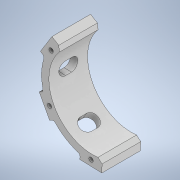
# Autodesk Inventor part: end_holder_3
Saved by Autodesk Inventor 2020 (Build 240168000, 168)
## iProperties
Created: 2020-11-16
Part Number: end_holder_3
Material: Generic
Document SubType Name: Modeling
Designer: Shuang Peng
Density: 1 g/cm^3
Appearance: Default
Author: Shuang Peng
Autodesk Inventor part; units mm, degrees
ref_plane "Work Plane1" through (0, 0, 0) normal (0, 0, 1) x (1, 0, 0)
sketch "Sketch1" plane through (0, 0, 0) normal (0, 0, 1) x (1, 0, 0)
  line L0 (-114.7595, -23.8164) -> (-86.516, -0.3214) projected
  arc A0 (-83.238, -1.9261) -> (-86.516, -0.3214) centre (-85.2369, -1.8589) ccw projected
  arc A1 (-83.238, -1.9261) -> (-80.4978, -22.1613) centre (-22.2724, -3.9734) ccw projected
  arc A2 (-84.3159, -27.354) -> (-80.4978, -22.1613) centre (-84.3159, -23.354) ccw projected
  line L1 (-84.3159, -27.354) -> (-113.4805, -27.354) projected
  arc A3 (-114.7595, -23.8164) -> (-113.4805, -27.354) centre (-113.4805, -25.354) ccw projected
  circle A4 centre (71.296, -16.8454) radius 1.5 projected
  circle A5 centre (-18.8152, -59.8032) radius 1.5 projected
  circle A6 centre (-53.4562, -50.8504) radius 1.5 projected
  circle A7 centre (-60.8075, 36.5725) radius 1.5 projected
  circle A8 centre (-28.5162, 51.9811) radius 1.5 projected
  circle A9 centre (-9.173, 50.4079) radius 1.5 projected
  circle A10 centre (-44.8423, 47.6065) radius 1.5 projected
  circle A11 centre (-67.2628, -37.2117) radius 1.5 projected
  circle A12 centre (-38.1378, -57.9935) radius 1.5 projected
  circle A13 centre (45.81, -34.6909) radius 1.5 projected
  circle A14 centre (-22.2724, -3.9734) radius 24.5 projected
  line L2 (17.4995, 54.7179) -> (28.6687, 48.4472) projected
  line L3 (8.4026, 48.2499) -> (17.4995, 54.7179) projected
  arc A15 (6.5013, 48.0227) -> (8.4026, 48.2499) centre (7.2436, 49.8798) ccw projected
  line L4 (-7.3529, 53.5603) -> (6.5013, 48.0227) projected
  arc A16 (-7.3529, 53.5603) -> (-12.4241, 54.6417) centre (-22.2724, -3.9734) ccw projected
  line L5 (-12.5849, 53.6843) -> (-12.4241, 54.6417) projected
  arc A17 (-14.821, 52.0331) -> (-12.5849, 53.6843) centre (-14.5573, 54.0157) ccw projected
  arc A18 (-14.821, 52.0331) -> (-23.537, 52.5125) centre (-22.2724, -3.9734) ccw projected
  arc A19 (-25.5786, 54.3989) -> (-23.537, 52.5125) centre (-23.5818, 54.512) ccw projected
  line L6 (-25.6541, 55.7327) -> (-25.5786, 54.3989) projected
  arc A20 (-25.6541, 55.7327) -> (-31.8766, 55.0521) centre (-22.2724, -3.9734) ccw projected
  line L7 (-43.4677, 51.9463) -> (-31.8766, 55.0521) projected
  arc A21 (-43.4677, 51.9463) -> (-49.1968, 49.4245) centre (-22.2724, -3.9734) ccw projected
  line L8 (-48.5953, 48.2316) -> (-49.1968, 49.4245) projected
  arc A22 (-49.4201, 45.5771) -> (-48.5953, 48.2316) centre (-50.3811, 47.3311) ccw projected
  arc A23 (-49.4201, 45.5771) -> (-56.7287, 40.804) centre (-22.2724, -3.9734) ccw projected
  arc A24 (-59.4908, 41.1159) -> (-56.7287, 40.804) centre (-57.9484, 42.389) ccw projected
  line L9 (-60.1088, 41.8646) -> (-59.4908, 41.1159) projected
  arc A25 (-60.1088, 41.8646) -> (-63.9599, 38.3925) centre (-22.2724, -3.9734) ccw projected
  line L10 (-73.8637, 25.8129) -> (-63.9599, 38.3925) projected
  line L11 (-73.8637, 25.8129) -> (-144.5637, -33.0004) projected
  arc A26 (-144.5637, -33.0004) -> (-146.1648, -34.4172) centre (-122.1805, -59.9075) ccw projected
  arc A27 (-148.5912, -34.6592) -> (-146.1648, -34.4172) centre (-147.5353, -32.9607) ccw projected
  line L12 (-148.5912, -34.6592) -> (-150.0693, -33.7404) projected
  line L13 (-150.0693, -33.7404) -> (-157.9882, -46.4797) projected
  line L14 (-157.9882, -46.4797) -> (-156.5102, -47.3985) projected
  arc A28 (-155.6533, -49.6815) -> (-156.5102, -47.3985) centre (-157.566, -49.0971) ccw projected
  arc A29 (-155.6533, -49.6815) -> (-156.2478, -67.9334) centre (-122.1805, -59.9075) ccw projected
  arc A30 (-157.2515, -70.1557) -> (-156.2478, -67.9334) centre (-158.1945, -68.392) ccw projected
  line L15 (-157.2515, -70.1557) -> (-158.7862, -70.9764) projected
  line L16 (-158.7862, -70.9764) -> (-151.7131, -84.204) projected
  line L17 (-151.7131, -84.204) -> (-150.1784, -83.3834) projected
  arc A31 (-147.7729, -83.7828) -> (-150.1784, -83.3834) centre (-149.2353, -85.1471) ccw projected
  arc A32 (-147.7729, -83.7828) -> (-132.2635, -93.4236) centre (-122.1805, -59.9075) ccw projected
  arc A33 (-130.8408, -95.404) -> (-132.2635, -93.4236) centre (-132.8397, -95.3388) ccw projected
  line L18 (-130.8408, -95.404) -> (-130.8974, -97.1434) projected
  line L19 (-130.8974, -97.1434) -> (-115.9054, -97.6318) projected
  line L20 (-115.9054, -97.6318) -> (-115.8487, -95.8923) projected
  arc A34 (-114.3001, -94.0088) -> (-115.8487, -95.8923) centre (-113.8498, -95.9574) ccw projected
  arc A35 (-114.3001, -94.0088) -> (-111.5272, -93.2468) centre (-122.1805, -59.9075) ccw projected
  line L21 (-111.5272, -93.2468) -> (-17.5702, -63.2237) projected
  line L22 (-1.8974, -59.9532) -> (-17.5702, -63.2237) projected
  line L23 (-3.6226, -55.2133) -> (-1.8974, -59.9532) projected
  arc A36 (-2.4006, -52.6404) -> (-3.6226, -55.2133) centre (-1.7432, -54.5293) ccw projected
  line L24 (40.7711, -37.6143) -> (-2.4006, -52.6404) projected
  arc A37 (41.7759, -37.5336) -> (40.7711, -37.6143) centre (41.4286, -39.5032) ccw projected
  line L25 (49.1414, -38.8323) -> (41.7759, -37.5336) projected
  line L26 (49.5371, -36.5883) -> (49.1414, -38.8323) projected
  arc A38 (51.1536, -34.967) -> (49.5371, -36.5883) centre (51.5067, -36.9355) ccw projected
  arc A39 (51.1536, -34.967) -> (69.7278, -21.9611) centre (46.3856, -8.3913) ccw projected
  arc A40 (71.8042, -20.9967) -> (69.7278, -21.9611) centre (71.4569, -22.9663) ccw projected
  line L27 (74.0482, -21.3924) -> (71.8042, -20.9967) projected
  line L28 (78.128, 1.745) -> (74.0482, -21.3924) projected
  line L29 (78.128, 1.745) -> (69.8258, 3.2089) projected
  arc A41 (28.6687, 48.4472) -> (69.8258, 3.2089) centre (78.5082, 52.4493) ccw projected
  circle A42 centre (46.3856, -8.3913) radius 8 projected
  circle A43 centre (24.8362, 42.9855) radius 2.1 projected
  circle A44 centre (69.0444, -1.2227) radius 2.1 projected
  circle A45 centre (32.9741, 22.501) radius 2.1 projected
  circle A46 centre (48.56, 6.9152) radius 2.1 projected
  line L30 (61.5225, -11.0604) -> (64.993, -11.6723) projected
  arc A47 (66.5678, -14.1946) -> (64.993, -11.6723) centre (64.6457, -13.6419) ccw projected
  arc A48 (55.6053, -27.2592) -> (66.5678, -14.1946) centre (46.3856, -8.3913) ccw projected
  arc A49 (52.8479, -26.1463) -> (55.6053, -27.2592) centre (54.7273, -25.4622) ccw projected
  line L31 (52.8479, -26.1463) -> (51.6426, -22.8348) projected
  arc A50 (52.6012, -20.3753) -> (51.6426, -22.8348) centre (53.522, -22.1507) ccw projected
  arc A51 (52.6012, -20.3753) -> (59.2669, -12.4314) centre (46.3856, -8.3913) ccw projected
  arc A52 (61.5225, -11.0604) -> (59.2669, -12.4314) centre (61.1752, -13.03) ccw projected
  arc A53 (28.8077, -30.3754) -> (33.319, -18.6649) centre (-22.2724, -3.9734) ccw projected
  arc A54 (36.6892, -17.7843) -> (33.319, -18.6649) centre (35.2527, -19.1759) ccw projected
  arc A55 (36.6892, -17.7843) -> (42.4768, -21.313) centre (46.3856, -8.3913) ccw projected
  arc A56 (43.0588, -24.8558) -> (42.4768, -21.313) centre (41.8977, -23.2274) ccw projected
  line L32 (43.0588, -24.8558) -> (31.7455, -32.9222) projected
  arc A57 (28.8077, -30.3754) -> (31.7455, -32.9222) centre (30.5844, -31.2938) ccw projected
  arc A58 (36.3695, 11.8712) -> (41.3146, 7.2953) centre (78.5082, 52.4493) ccw projected
  arc A59 (40.8614, 3.9267) -> (41.3146, 7.2953) centre (40.043, 5.7516) ccw projected
  arc A60 (40.8614, 3.9267) -> (37.576, 1.8381) centre (46.3856, -8.3913) ccw projected
  arc A61 (34.2864, 3.1052) -> (37.576, 1.8381) centre (36.2709, 3.3536) ccw projected
  arc A62 (34.2864, 3.1052) -> (32.9898, 9.9939) centre (-22.2724, -3.9734) ccw projected
  arc A63 (36.3695, 11.8712) -> (32.9898, 9.9939) centre (34.9289, 10.4839) ccw projected
  circle A64 centre (-78.0027, -75.3364) radius 2 projected
  circle A65 centre (-110.6431, -14.2192) radius 2 projected
  circle A66 centre (-91.7471, -81.3441) radius 2 projected
  circle A67 centre (-123.1684, -22.4726) radius 2 projected
  circle A68 centre (-123.2712, -93.3897) radius 1.5 projected
  circle A69 centre (-150.6316, -42.2218) radius 1.5 projected
  circle A70 centre (-151.7223, -75.704) radius 1.5 projected
  circle A71 centre (-76.5892, -34.383) radius 2.05 projected
  circle A72 centre (-93.5857, -34.7301) radius 2.05 projected
  circle A73 centre (-85.7696, -48.6911) radius 2.05 projected
  line L33 (25.2192, -8.9275) -> (12.7605, -6.9639) projected
  arc A74 (10.2276, -3.9982) -> (12.7605, -6.9639) centre (13.2276, -4.0005) ccw projected
  arc A75 (10.2276, -3.9982) -> (9.854, 0.9403) centre (-22.2724, -3.9734) ccw projected
  arc A76 (12.117, 4.3104) -> (9.854, 0.9403) centre (12.8195, 1.3938) ccw projected
  line L34 (12.117, 4.3104) -> (24.3016, 7.2454) projected
  arc A77 (27.9589, 4.8477) -> (24.3016, 7.2454) centre (25.0042, 4.3289) ccw projected
  arc A78 (28.6837, -6.0885) -> (27.9589, 4.8477) centre (-22.2724, -3.9734) ccw projected
  arc A79 (25.2192, -8.9275) -> (28.6837, -6.0885) centre (25.6863, -5.9641) ccw projected
  line L35 (18.5933, -28.9733) -> (7.9021, -22.4328) projected
  arc A80 (6.7854, -18.53) -> (7.9021, -22.4328) centre (9.4676, -19.8737) ccw projected
  arc A81 (6.7854, -18.53) -> (8.6598, -13.9459) centre (-22.2724, -3.9734) ccw projected
  arc A82 (11.9821, -11.903) -> (8.6598, -13.9459) centre (11.515, -14.8664) ccw projected
  line L36 (11.9821, -11.903) -> (24.4408, -13.8666) projected
  arc A83 (26.8641, -17.6335) -> (24.4408, -13.8666) centre (23.9738, -16.83) ccw projected
  arc A84 (22.8108, -27.8167) -> (26.8641, -17.6335) centre (-22.2724, -3.9734) ccw projected
  arc A85 (18.5933, -28.9733) -> (22.8108, -27.8167) centre (20.1588, -26.4142) ccw projected
  line L37 (-4.4447, -43.3488) -> (-7.3459, -35.8081) projected
  arc A86 (-6.0439, -32.1316) -> (-7.3459, -35.8081) centre (-4.5459, -34.7308) ccw projected
  arc A87 (-6.0439, -32.1316) -> (-1.9539, -29.3388) centre (-22.2724, -3.9734) ccw projected
  arc A88 (2.0962, -29.6136) -> (-1.9539, -29.3388) centre (-0.0783, -31.6803) ccw projected
  line L38 (2.0962, -29.6136) -> (7.6236, -35.4294) projected
  arc A89 (7.3609, -39.808) -> (7.6236, -35.4294) centre (5.449, -37.4961) ccw projected
  arc A90 (-0.2222, -44.9128) -> (7.3609, -39.808) centre (-22.2724, -3.9734) ccw projected
  arc A91 (-4.4447, -43.3488) -> (-0.2222, -44.9128) centre (-1.6448, -42.2715) ccw projected
  line L39 (-23.3755, -47.3558) -> (-23.1715, -39.3349) projected
  arc A92 (-20.35, -36.4165) -> (-23.1715, -39.3349) centre (-20.1725, -39.4112) ccw projected
  arc A93 (-20.35, -36.4165) -> (-15.4428, -35.7477) centre (-22.2724, -3.9734) ccw projected
  arc A94 (-12.0124, -37.6034) -> (-15.4428, -35.7477) centre (-14.8123, -38.6807) ccw projected
  line L40 (-12.0124, -37.6034) -> (-9.1112, -45.1441) projected
  arc A95 (-11.1966, -49.135) -> (-9.1112, -45.1441) centre (-11.9112, -46.2214) ccw projected
  arc A96 (-20.2457, -50.4292) -> (-11.1966, -49.135) centre (-22.2724, -3.9734) ccw projected
  arc A97 (-23.3755, -47.3558) -> (-20.2457, -50.4292) centre (-20.3765, -47.432) ccw projected
  line L41 (-50.3087, -42.6252) -> (-42.3788, -32.8175) projected
  arc A98 (-38.5439, -32.1067) -> (-42.3788, -32.8175) centre (-40.0459, -34.7037) ccw projected
  arc A99 (-38.5439, -32.1067) -> (-34.0803, -34.2525) centre (-22.2724, -3.9734) ccw projected
  arc A100 (-32.2932, -37.8973) -> (-34.0803, -34.2525) centre (-35.1703, -37.0474) ccw projected
  line L42 (-32.2932, -37.8973) -> (-35.8437, -49.917) projected
  arc A101 (-39.7488, -51.8855) -> (-35.8437, -49.917) centre (-38.7208, -49.0672) ccw projected
  arc A102 (-49.5823, -47.0451) -> (-39.7488, -51.8855) centre (-22.2724, -3.9734) ccw projected
  arc A103 (-50.3087, -42.6252) -> (-49.5823, -47.0451) centre (-47.9758, -44.5114) ccw projected
  line L43 (-64.3558, -26.8641) -> (-53.346, -20.8755) projected
  arc A104 (-49.4077, -21.8598) -> (-53.346, -20.8755) centre (-51.9125, -23.5108) ccw projected
  arc A105 (-49.4077, -21.8598) -> (-46.3749, -25.7752) centre (-22.2724, -3.9734) ccw projected
  arc A106 (-46.2669, -29.6738) -> (-46.3749, -25.7752) centre (-48.5998, -27.7876) ccw projected
  line L44 (-46.2669, -29.6738) -> (-54.1968, -39.4816) projected
  arc A107 (-58.6707, -39.6968) -> (-54.1968, -39.4816) centre (-56.5296, -37.5954) ccw projected
  arc A108 (-65.463, -31.0949) -> (-58.6707, -39.6968) centre (-22.2724, -3.9734) ccw projected
  arc A109 (-64.3558, -26.8641) -> (-65.463, -31.0949) centre (-62.9223, -29.4995) ccw projected
  line L45 (-65.2864, 0.2751) -> (-57.3053, -0.9828) projected
  arc A110 (-54.7724, -3.9485) -> (-57.3053, -0.9828) centre (-57.7724, -3.9462) ccw projected
  arc A111 (-54.7724, -3.9485) -> (-54.3988, -8.887) centre (-22.2724, -3.9734) ccw projected
  arc A112 (-56.6618, -12.2571) -> (-54.3988, -8.887) centre (-57.3643, -9.3405) ccw projected
  line L46 (-56.6618, -12.2571) -> (-64.4621, -14.1361) projected
  arc A113 (-68.1227, -11.7192) -> (-64.4621, -14.1361) centre (-65.1646, -11.2195) ccw projected
  arc A114 (-68.7521, -2.5997) -> (-68.1227, -11.7192) centre (-22.2724, -3.9734) ccw projected
  arc A115 (-65.2864, 0.2751) -> (-68.7521, -2.5997) centre (-65.7534, -2.6883) ccw projected
  line L47 (-59.2911, 18.6731) -> (-52.4469, 14.4861) projected
  arc A116 (-51.3302, 10.5833) -> (-52.4469, 14.4861) centre (-54.0124, 11.927) ccw projected
  arc A117 (-51.3302, 10.5833) -> (-53.2046, 5.9991) centre (-22.2724, -3.9734) ccw projected
  arc A118 (-56.5269, 3.9563) -> (-53.2046, 5.9991) centre (-56.0599, 6.9197) ccw projected
  line L48 (-56.5269, 3.9563) -> (-64.5079, 5.2141) projected
  arc A119 (-66.9215, 9.0155) -> (-64.5079, 5.2141) centre (-64.0409, 8.1775) ccw projected
  arc A120 (-63.5177, 17.4994) -> (-66.9215, 9.0155) centre (-22.2724, -3.9734) ccw projected
  arc A121 (-59.2911, 18.6731) -> (-63.5177, 17.4994) centre (-60.8567, 16.114) ccw projected
  line L49 (-41.7278, 39.6327) -> (-37.199, 27.8613) projected
  arc A122 (-38.5009, 24.1849) -> (-37.199, 27.8613) centre (-39.9989, 26.7841) ccw projected
  arc A123 (-38.5009, 24.1849) -> (-42.5909, 21.3921) centre (-22.2724, -3.9734) ccw projected
  arc A124 (-46.641, 21.6668) -> (-42.5909, 21.3921) centre (-44.4665, 23.7336) ccw projected
  line L50 (-46.641, 21.6668) -> (-55.2752, 30.7515) projected
  arc A125 (-55.0274, 35.1177) -> (-55.2752, 30.7515) centre (-53.1006, 32.8182) ccw projected
  arc A126 (-45.9187, 41.2135) -> (-55.0274, 35.1177) centre (-22.2724, -3.9734) ccw projected
  arc A127 (-41.7278, 39.6327) -> (-45.9187, 41.2135) centre (-44.5277, 38.5555) ccw projected
  line L51 (-21.0547, 43.9173) -> (-21.3733, 31.3882) projected
  arc A128 (-24.1948, 28.4697) -> (-21.3733, 31.3882) centre (-24.3723, 31.4645) ccw projected
  arc A129 (-24.1948, 28.4697) -> (-29.1021, 27.8009) centre (-22.2724, -3.9734) ccw projected
  arc A130 (-32.5324, 29.6567) -> (-29.1021, 27.8009) centre (-29.7325, 30.7339) ccw projected
  line L52 (-32.5324, 29.6567) -> (-37.0613, 41.4281) projected
  arc A131 (-35.0106, 45.4102) -> (-37.0613, 41.4281) centre (-34.2613, 42.5053) ccw projected
  arc A132 (-24.1651, 46.9915) -> (-35.0106, 45.4102) centre (-22.2724, -3.9734) ccw projected
  arc A133 (-21.0547, 43.9173) -> (-24.1651, 46.9915) centre (-24.0537, 43.9936) ccw projected
  line L53 (5.7638, 34.6785) -> (-2.166, 24.8708) projected
  arc A134 (-6.0009, 24.16) -> (-2.166, 24.8708) centre (-4.4989, 26.757) ccw projected
  arc A135 (-6.0009, 24.16) -> (-10.4645, 26.3057) centre (-22.2724, -3.9734) ccw projected
  arc A136 (-12.2517, 29.9506) -> (-10.4645, 26.3057) centre (-9.3746, 29.1007) ccw projected
  line L54 (-12.2517, 29.9506) -> (-8.7012, 41.9703) projected
  arc A137 (-4.796, 43.9388) -> (-8.7012, 41.9703) centre (-5.8241, 41.1205) ccw projected
  arc A138 (5.0374, 39.0984) -> (-4.796, 43.9388) centre (-22.2724, -3.9734) ccw projected
  arc A139 (5.7638, 34.6785) -> (5.0374, 39.0984) centre (3.431, 36.5647) ccw projected
  circle A140 centre (18.7379, 18.9865) radius 2.05 projected
  circle A141 centre (5.6495, 11.6589) radius 2.05 projected
  arc A142 (-88.373, -68.9659) -> (-87.2274, -61.7195) centre (-122.1805, -59.9075) ccw projected
  arc A143 (-84.7539, -56.3391) -> (-87.2274, -61.7195) centre (-79.2381, -62.1337) ccw projected
  line L55 (-84.7539, -56.3391) -> (-72.896, -45.0519) projected
  arc A144 (-67.1926, -45.2429) -> (-72.896, -45.0519) centre (-70.1382, -47.9491) ccw projected
  arc A145 (-67.1926, -45.2429) -> (-52.2157, -57.1184) centre (-22.2724, -3.9734) ccw projected
  arc A146 (-52.5887, -60.766) -> (-52.2157, -57.1184) centre (-53.1975, -58.8609) ccw projected
  line L56 (-52.5887, -60.766) -> (-85.8324, -71.3887) projected
  arc A147 (-88.373, -68.9659) -> (-85.8324, -71.3887) centre (-86.4412, -69.4836) ccw projected
  arc A148 (-119.4703, -38.0751) -> (-123.464, -37.945) centre (-121.4642, -37.9192) ccw projected
  arc A149 (-100.218, -58.6239) -> (-119.4703, -38.0751) centre (-122.1805, -59.9075) ccw projected
  arc A150 (-100.3481, -62.6177) -> (-100.218, -58.6239) centre (-100.1921, -60.6238) ccw projected
  arc A151 (-120.8969, -81.87) -> (-100.3481, -62.6177) centre (-122.1805, -59.9075) ccw projected
  arc A152 (-124.8907, -81.7399) -> (-120.8969, -81.87) centre (-122.8968, -81.8958) ccw projected
  arc A153 (-144.143, -61.191) -> (-124.8907, -81.7399) centre (-122.1805, -59.9075) ccw projected
  arc A154 (-144.0129, -57.1973) -> (-144.143, -61.191) centre (-144.1688, -59.1912) ccw projected
  arc A155 (-123.464, -37.945) -> (-144.0129, -57.1973) centre (-122.1805, -59.9075) ccw projected
  circle A156 centre (-122.1805, -59.9075) radius 30
  line L57 (-148.5912, -34.6592) -> (-142.8906, -38.2028)
  line L58 (-115.8487, -95.8923) -> (-115.6302, -89.1836)
  point P0 (0, 0)
  dimension "d0" = 60
  constraints: 4 end point, 2 collinear, 2 point on circle, 1 centre point, 1 coincident
  measures "d0" diameter of A156
ref_plane "Work Plane2" through (-195.3769, -166.2263, 26.5) normal (0, 0, -1) x (-0.0309, 0.9995, 0)
extrude "Extrusion1" add sketch "Sketch1" along normal up to surface (26.5 mm away) contours L20 L19 L18 A33 A32 A31 L17 L16 L15 A30 A29 A28 L14 L13 L12 L57 A156 L58
chamfer "Chamfer1" distance 3 angle 45 2 edges at (-142.8906, -38.2028, 13.25) (-115.6302, -89.1836, 13.25)
ref_plane "Work Plane3" through (-157.9882, -46.4797, 0) normal (0.9995, -0.0326, 0) x (0, 0, 1)
sketch "Sketch2" plane through (-157.9882, -46.4797, 0) normal (0.9995, -0.0326, 0) x (0, 0, 1)
  line L0 (26.5, 3.124) -> (26.5, 21.3856) projected
  line L1 (0, 3.124) -> (26.5, 3.124) projected
  line L2 (0, 3.124) -> (0, 21.3856) projected
  line L3 (0, 21.3856) -> (26.5, 21.3856) projected
  line L4 (0, 23.6394) -> (0, 21.3856) projected
  line L5 (26.5, 3.124) -> (0, 21.3856)
  line L6 (0, 21.3856) -> (26.5, 21.3856)
  line L7 (26.5, 23.6394) -> (26.5, 21.3856) projected
  line L8 (26.5, 21.3856) -> (0, 3.124)
  line L9 (15.25, 12.2548) -> (11.25, 12.2548) construction
  line L10 (15.25, 16.7548) -> (11.25, 16.7548)
  line L11 (11.25, 7.7548) -> (15.25, 7.7548)
  arc A0 (15.25, 7.7548) -> (15.25, 16.7548) centre (15.25, 12.2548) ccw
  arc A1 (11.25, 16.7548) -> (11.25, 7.7548) centre (11.25, 12.2548) ccw
  point P0 (0, -51.5989)
  point P1 (13.25, 12.2548)
  dimension "d6" = 2
  dimension "d7" = 9
  constraints: 14 end point, 4 point on circle, 4 tangent, 2 centre point, 2 midpoint, 1 horizontal, 1 parallel, 1 perpendicular
  measures "d6" distance of point (13.25, 12.255) L9.end
  measures "d7" diameter of A1
extrude "Extrusion2" cut sketch "Sketch2" along normal blind 10 contours A0 L11 A1 L8 L5 | L5 L8 A0 | L8 L5 A1 L10 A0 | A1 L5 L8
ref_plane "Work Plane4" through (-114.5435, -55.8238, 26.5) normal (-0.4715, 0.8818, 0) x (0, 0, 1)
mirror "Mirror1" about plane through (-114.5435, -55.8238, 26.5) normal (-0.4715, 0.8818, 0) of "Extrusion2"
body "Solid1"
